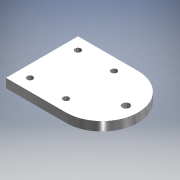
# Autodesk Inventor part: steeringPlate
Saved by Autodesk Inventor 2018 (Build 220112000, 112)
## iProperties
Created: 2018-08-03
Part Number: steeringPlate
Material: Aluminum 6061
Document SubType Name: Modeling
Designer: Cole Tucker
Density: 2.7 g/cm^3
Appearance: Aluminum - Flat
Author: Cole Tucker
Autodesk Inventor part; units mm, degrees
ref_plane "YZ Plane" through (0, 0, 0) normal (1, 0, 0) x (0, 1, 0)
ref_plane "XZ Plane" through (0, 0, 0) normal (0, 1, 0) x (-1, 0, 0)
ref_plane "XY Plane" through (0, 0, 0) normal (0, 0, 1) x (1, 0, 0)
sketch "Sketch1" plane through (0, 0, 0) normal (0, 1, 0) x (-1, 0, 0)
  line L0 (0, 0) -> (-101.6, 0)
  line L1 (-101.6, 0) -> (-101.6, -76.2)
  line L2 (-101.6, -76.2) -> (0, -76.2)
  line L3 (0, -76.2) -> (0, 0)
  line L4 (-76.2, 0) -> (-76.2, -76.2) construction
  line L5 (-76.2, 0) -> (-76.2, -12.7) construction
  line L6 (-76.2, -76.2) -> (-76.2, -63.5) construction
  line L7 (-76.2, -63.5) -> (0, -63.5) construction
  line L8 (-76.2, -12.7) -> (0, -12.7) construction
  circle A0 centre (-12.7, -12.7) radius 3.175
  circle A1 centre (-50.8, -12.7) radius 3.175
  circle A2 centre (-12.7, -63.5) radius 3.175
  circle A3 centre (-50.8, -63.5) radius 3.175
  line L9 (-76.2, -38.1) -> (-101.6, -38.1) construction
  circle A4 centre (-88.9, -38.1) radius 3.9687
  dimension "d0" = 101.6
  dimension "d1" = 76.2
  dimension "d2" = 76.2
  dimension "d3" = 12.7
  dimension "d4" = 12.7
  dimension "d5" = 6.35
  dimension "d7" = 6.35
  dimension "d8" = 6.35
  dimension "d10" = 6.35
  dimension "d11" = 12.7
  dimension "d12" = 12.7
  dimension "d15" = 50.8
  dimension "d16" = 50.8
  dimension "d17" = 7.9375
  constraints: 20 end point, 10 point on line, 5 centre point, 4 perpendicular, 3 midpoint, 2 parallel, 1 horizontal
  measures "d0" distance of L2.end L1.end
  measures "d1" distance of L1.end L0.end
  measures "d2" distance between parallel lines of L3 L4
  measures "d3" distance of L4.start L5.end
  measures "d4" distance of L4.end L6.end
  measures "d5" diameter of A0
  measures "d7" diameter of A1
  measures "d8" diameter of A2
  measures "d10" diameter of A3
  measures "d11" distance from line of L3 A0.centre
  measures "d12" distance from line of L3 A2.centre
  measures "d15" distance from line of L3 A1.centre
  measures "d16" distance from line of L3 A3.centre
  measures "d17" diameter of A4
extrude "Extrusion1" add sketch "Sketch1" along normal blind 9.525
fillet "Fillet1" radius 38.1 2 edges at (101.6, 4.7625, 0) (101.6, 4.7625, -76.2)
equation "\"d12\" = d11"
equation "\"d16\" = d15"
body "Solid1"
